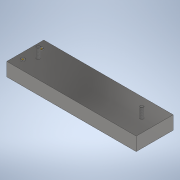
# Autodesk Inventor part: resistencia_cuarzo_250-300W
Saved by Autodesk Inventor 2021 (Build 250183000, 183)
## iProperties
Created: 2021-04-16
Part Number: resistencia_cuarzo_250-300W
Material: Genérico
Document SubType Name: Modeling
Designer: Leonardo Fabio Mercado Benítez
Density: 1 g/cm^3
Appearance: Valor por defecto
Categories: <MemberInstance><Categories><Category DisplayName="" Mnemonic="CABLEANDHARNESS" InternalName="e4a7e005-5e42-4d16-b293-125e7f0d0512"><Category DisplayName="" Mnemonic="CONNECTORS" InternalName="6f634eba-a678-4820-a31d-2c2d5ee6728e"><CategoryParameter DisplayName="" Mnemonic="REFDES" InternalName="c3740e8c-60ab-4d5d-8584-52b73222f2f0"/><Category DisplayName="" Mnemonic="DISCRETEWIRE" InternalName="9a3407de-09b2-4cdb-8c40-9708d5144a28"/></Category></Category></Categories><FamilyTemplate><FamilyTemplateParameters></FamilyTemplateParameters></FamilyTemplate><CategoryParameterMap><ParamToTemplateMap><ParamToTemplate CategoryParameter="//CategoryParameter[@InternalName='c3740e8c-60ab-4d5d-8584-52b73222f2f0']" ConstantValue=""/></ParamToTemplateMap></CategoryParameterMap></MemberInstance>
Author: Leonardo Fabio Mercado Benítez
Autodesk Inventor part; units mm, degrees
ref_plane "YZ Plane" through (0, 0, 0) normal (1, 0, 0) x (0, 1, 0)
ref_plane "XZ Plane" through (0, 0, 0) normal (0, 1, 0) x (-1, 0, 0)
ref_plane "XY Plane" through (0, 0, 0) normal (0, 0, 1) x (1, 0, 0)
sketch "Boceto1" plane through (0, 0, 0) normal (0, 1, 0) x (-1, 0, 0)
  line L0 (-122.5, 35) -> (122.5, 35)
  line L1 (122.5, 35) -> (122.5, -35)
  line L2 (122.5, -35) -> (-122.5, -35)
  line L3 (-122.5, -35) -> (-122.5, 35)
  line L4 (-122.5, 35) -> (122.5, -35) construction
  line L5 (122.5, 35) -> (-122.5, -35) construction
  point P0 (0, 0)
  dimension "d0" = 245
  dimension "d1" = 70
  constraints: 12 end point, 2 midpoint, 2 parallel, 1 horizontal, 1 perpendicular
  measures "d0" distance of L1.end L2.end
  measures "d1" distance of L0.end L1.end
extrude "Extrusión1" add sketch "Boceto1" along normal blind 25.4
sketch "Boceto2" plane through (0, 0, 0) normal (0, -1, 0) x (1, 0, 0)
  line L0 (-109.8, 33.98) -> (109.8, 33.98)
  line L1 (109.8, -33.98) -> (-109.8, -33.98)
  line L2 (-109.8, -33.98) -> (-109.8, 33.98)
  line L3 (109.8, 33.98) -> (109.8, -33.98)
  line L4 (-122.5, -35) -> (-122.5, 35) projected
  line L5 (-122.5, 35) -> (122.5, 35) projected
  dimension "d8" = 12.7
  dimension "d9" = 1.02
  constraints: 8 end point
  measures "d8" distance between parallel lines of L4 L2
  measures "d9" distance between parallel lines of L5 L0
extrude "Extrusión2" cut sketch "Boceto2" against normal blind 24.38
sketch "Boceto3" plane through (-109.8, 0, 33.98) normal (1, 0, 0) x (0, 0, -1)
  line L0 (-1.02, 0) -> (-1.02, 25.4) construction
  line L1 (68.98, 0) -> (68.98, 25.4) construction
  circle A0 centre (6.5, 6.35) radius 4.7625
  line L2 (0, 0) -> (0, 24.38) projected
  line L3 (67.96, 0) -> (0, 0) projected
  circle A1 centre (17.5, 6.35) radius 4.7625
  circle A2 centre (28.5, 6.35) radius 4.7625
  circle A3 centre (39.5, 6.35) radius 4.7625
  circle A4 centre (50.5, 6.35) radius 4.7625
  circle A5 centre (61.5, 6.35) radius 4.7625
  point P0 (33.98, 0)
  dimension "d12" = 9.525
  dimension "d13" = 6.5
  dimension "d14" = 6.35
  dimension "d17" = 11
  constraints: 6 centre point, 1 horizontal, 10 other
  measures "d12" diameter of A0
  measures "d13" distance from line of L2 A0.centre
  measures "d14" distance from line of L3 A0.centre
  measures "d17" distance of A0.centre A1.centre
extrude "Extrusión3" add sketch "Boceto3" along normal up to surface (219.6 mm away)
sketch "Boceto4" plane through (0, 25.4, 0) normal (0, 1, 0) x (1, 0, 0)
  line L0 (-122.5, 35) -> (-73.5, 35) construction
  line L1 (-73.5, 35) -> (-73.5, -35) construction
  line L2 (-122.5, -35) -> (122.5, -35) construction
  line L3 (-122.5, -35) -> (-73.5, 35) construction
  line L4 (-122.5, 35) -> (-73.5, -35) construction
  line L5 (122.5, 35) -> (-122.5, 35) construction
  line L6 (122.5, 35) -> (73.5, 35) construction
  line L7 (73.5, 35) -> (73.5, -35) construction
  line L8 (73.5, -35) -> (122.5, 35) construction
  line L9 (73.5, 35) -> (122.5, -35) construction
  circle A0 centre (-98, 0) radius 3.175
  circle A1 centre (98, 0) radius 3.175
  point P0 (0, 0)
  dimension "d24" = 49
  dimension "d25" = 49
  dimension "d26" = 6.35
  dimension "d27" = 6.35
  constraints: 16 end point, 3 perpendicular, 3 point on line, 2 centre point, 2 midpoint
  measures "d24" distance of L0.start L0.end
  measures "d25" distance of L5.start L6.end
  measures "d26" diameter of A0
  measures "d27" diameter of A1
extrude "Extrusión4" add sketch "Boceto4" along normal blind 19.05
thread "Rosca1" size "1/4-20 UNC" class "1A" standard "ANSI Unified Screw Threads" full length
thread "Rosca2" size "M7x1" class "6g" standard "ANSI Metric M Profile" full length
chamfer "Chaflán1" distance 0.5 angle 45 1 edges at (-101.175, 44.45, 0)
chamfer "Chaflán2" distance 0.5 angle 45 1 edges at (94.825, 44.45, 0)
sketch "Boceto5" plane through (0, 25.4, 0) normal (0, 1, 0) x (1, 0, 0)
  line L0 (-122.5, -35) -> (122.5, -35) construction
  line L1 (-109.8, -35) -> (-109.8, 35.0447) construction
  line L2 (-122.5, 35) -> (-122.5, -35) construction
  line L3 (-109.8, -35) -> (-109.8, -17.489) construction
  line L4 (-109.8, -11.7175) -> (-109.8, -21.2425) construction
  line L5 (-109.8, 35.0447) -> (-109.8, 17.5337) construction
  line L6 (-109.8, 33.98) -> (-109.8, -33.98) construction
  circle A0 centre (-109.8, -17.489) radius 3.175
  circle A1 centre (-109.8, 17.5337) radius 3.175
  circle A2 centre (-109.8, -17.489) radius 3.685
  circle A3 centre (-109.8, 17.5337) radius 3.685
  point P0 (0, 0)
  dimension "d40" = 12.7
  dimension "d41" = 17.511
  dimension "d42" = 17.511
  dimension "d43" = 6.35
  dimension "d44" = 6.35
  dimension "d45" = 7.37
  dimension "d46" = 7.37
  constraints: 6 end point, 4 centre point, 4 coincident, 3 point on line, 1 vertical
  measures "d40" distance between parallel lines of L2 L1
  measures "d41" distance of L1.start L3.end
  measures "d42" distance of L1.end L5.end
  measures "d43" diameter of A0
  measures "d44" diameter of A1
  measures "d45" diameter of A2
  measures "d46" diameter of A3
extrude "Extrusión5" add sketch "Boceto5" along normal blind 2
chamfer "Chaflán3" distance 0.5 angle 45 2 edges at (-113.485, 27.4, -17.5337) (-113.485, 27.4, 17.489)
sketch "Boceto6" plane through (-109.8, 25.4, 17.489) normal (0, 1, 0) x (1, 0, 0)
  circle A0 centre (0, 0) radius 3.175 projected
sketch "Boceto7" plane through (-109.8, 25.4, -17.5337) normal (0, 1, 0) x (1, 0, 0)
  circle A0 centre (0, 0) radius 3.175 projected
